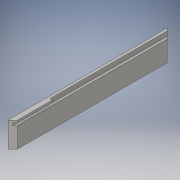
# Autodesk Inventor part: Base Runner Side
Saved by Autodesk Inventor 2016 (Build 200138000, 138)
## iProperties
Created: 2017-11-04
Part Number: Base Runner Side
Material: Generic
Document SubType Name: Modeling
Designer: mathaetaes
Density: 1 g/cm^3
Appearance: Default
Author: mathaetaes
Autodesk Inventor part; units mm, degrees
ref_plane "YZ Plane" through (0, 0, 0) normal (1, 0, 0) x (0, 1, 0)
ref_plane "XZ Plane" through (0, 0, 0) normal (0, 1, 0) x (-1, 0, 0)
ref_plane "XY Plane" through (0, 0, 0) normal (0, 0, 1) x (1, 0, 0)
sketch "Sketch1" plane through (0, 0, 0) normal (1, 0, 0) x (0, 1, 0)
  line L0 (64.7557, 327.0674) -> (-36.8443, 327.0674)
  line L1 (-36.8443, 327.0674) -> (-36.8443, -314.2826)
  line L2 (-36.8443, -314.2826) -> (64.7557, -314.2826)
  line L3 (64.7557, -314.2826) -> (64.7557, 327.0674)
  dimension "d2" = 641.35
  dimension "d3" = 101.6
  constraints: 8 end point, 2 parallel, 1 horizontal, 1 perpendicular
  measures "d2" distance of L0.end L1.end
  measures "d3" distance of L1.end L2.end
extrude "Board" add sketch "Sketch1" along normal blind 19.05
sketch "Sketch8" plane through (19.05, 0, 0) normal (1, 0, 0) x (0, 0, -1)
  line L0 (-327.0674, 55.2307) -> (314.2826, 55.2307)
  line L1 (314.2826, 55.2307) -> (314.2826, 45.7057)
  line L2 (314.2826, 45.7057) -> (-327.0674, 45.7057)
  line L3 (-327.0674, 45.7057) -> (-327.0674, 55.2307)
  line L4 (-327.0674, 64.7557) -> (-327.0674, -36.8443) projected
  line L5 (314.2826, -36.8443) -> (314.2826, 64.7557) projected
  line L6 (314.2826, 64.7557) -> (-327.0674, 64.7557) projected
  point P0 (0, 0)
  dimension "d22" = 9.525
  dimension "d23" = 9.525
  constraints: 8 end point, 2 collinear, 2 parallel, 1 horizontal, 1 perpendicular
  measures "d22" distance of L0.end L1.end
  measures "d23" distance between parallel lines of L6 L0
extrude "Lenghtwise Dado for Base" cut sketch "Sketch8" against normal blind 9.525 contours L0 L1 L2 L3
sketch "Sketch 9" plane through (0, 64.7557, 327.0674) normal (0, 1, 0) x (1, 0, 0)
  line L0 (19.05, 158.75) -> (9.525, 158.75)
  line L1 (9.525, 158.75) -> (9.525, 641.35)
  line L2 (9.525, 641.35) -> (19.05, 641.35)
  line L3 (19.05, 641.35) -> (19.05, 158.75)
  line L4 (19.05, 641.35) -> (19.05, 0) projected
  line L5 (0, 641.35) -> (19.05, 641.35) projected
  point P0 (0, 327.0674)
  dimension "d26" = 482.6
  dimension "d27" = 9.525
  constraints: 8 end point, 2 collinear, 2 parallel, 1 horizontal, 1 perpendicular
  measures "d26" distance of L2.end L0.start
  measures "d27" distance of L1.end L2.end
extrude "Lengthwise stop dado for Sides" cut sketch "Sketch 9" against normal blind 9.525
sketch "Sketch7" plane through (0, 64.7557, 327.0674) normal (0, 1, 0) x (1, 0, 0)
  line L0 (0, 641.35) -> (19.05, 641.35) projected
  line L1 (0, 641.35) -> (25.7054, 641.35) construction
  line L2 (0, 0) -> (19.05, 19.05)
  line L3 (19.05, 0) -> (19.05, 641.35) projected
  line L4 (19.05, 19.05) -> (19.05, 0)
  line L5 (0, 641.35) -> (19.05, 641.35)
  line L6 (0, 641.35) -> (19.05, 622.3)
  line L7 (19.05, 641.35) -> (19.05, 622.3)
  line L8 (0, 0) -> (19.05, 0) projected
  line L9 (19.05, 0) -> (0, 0)
  point P0 (0, 327.0674)
  dimension "d20" = 19.05
  dimension "d21" = 19.05
  constraints: 14 end point, 3 collinear, 2 horizontal, 2 point on line
  measures "d20" distance of L0.end L6.end
  measures "d21" distance of L3.start L2.end
extrude "45deg Mitre Cuts" cut sketch "Sketch7" against normal blind 101.6
equation "\"d18\" = d3"
body "Solid1"
